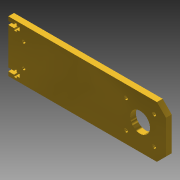
# Autodesk Inventor part: tiltColumnStepperSide02_RB01
Saved by Autodesk Inventor 2013 (Build 170138000, 138)
## iProperties
Created: 2014-06-14
Part Number: tiltColumnStepperSide02_RB01
Material: Gold
Document SubType Name: Modeling
Designer: Byron
Density: 19.3 g/cm^3
Mass: 1131.92 g
Surface Area: 227.905 cm^2
Volume: 58.6488 cm^3
Author: Byron
Autodesk Inventor part; units mm, degrees
ref_plane "YZ Plane" through (0, 0, 0) normal (1, 0, 0) x (0, 1, 0)
ref_plane "XZ Plane" through (0, 0, 0) normal (0, 1, 0) x (-1, 0, 0)
ref_plane "XY Plane" through (0, 0, 0) normal (0, 0, 1) x (1, 0, 0)
sketch "Sketch1" plane through (0, 0, 0) normal (0, 0, 1) x (1, 0, 0)
  circle A0 centre (15.5, -15.5) radius 2
  circle A1 centre (-15.5, -15.5) radius 2
  circle A2 centre (15.5, 15.5) radius 2
  circle A3 centre (-15.5, 15.5) radius 2
  line L0 (-21.15, 15.4985) -> (-15.4985, 21.15)
  line L1 (-15.4985, 21.15) -> (15.4985, 21.15)
  line L2 (15.4985, 21.15) -> (21.15, 15.4985)
  line L3 (21.15, 15.4985) -> (21.15, -15.4985)
  line L4 (21.15, -15.4985) -> (15.4985, -21.15)
  line L5 (15.4985, -21.15) -> (-15.4985, -21.15)
  line L6 (-15.4985, -21.15) -> (-21.15, -15.4985)
  line L7 (-21.15, -15.4985) -> (-21.15, 15.4985)
  line L8 (28.575, -18.574) -> (28.575, 18.574)
  line L9 (28.575, 18.574) -> (18.574, 28.575)
  line L10 (18.574, 28.575) -> (-18.574, 28.575)
  line L11 (-18.574, 28.575) -> (-28.575, 18.574)
  line L12 (-28.575, 18.574) -> (-28.575, -18.574)
  line L13 (-28.575, -18.574) -> (-18.574, -28.575)
  line L14 (-18.574, -28.575) -> (18.574, -28.575)
  line L15 (18.574, -28.575) -> (28.575, -18.574)
  line L16 (-18.574, -28.575) -> (-145.574, -28.575)
  line L17 (-145.574, -28.575) -> (-145.574, 28.575)
  line L18 (-145.574, 28.575) -> (-18.574, 28.575)
  line L19 (-18.574, 28.575) -> (-18.574, -28.575)
  circle A4 centre (0, 0) radius 11
  point P0 (0, 0)
  dimension "d0" = 127
  dimension "d1" = 57.15
  dimension "d2" = 57.15
  constraints: 40 end point, 5 centre point, 2 parallel, 1 horizontal, 1 perpendicular, 7 other
  measures "d0" distance of L17.end L18.end
  measures "d1" distance between parallel lines of L10 L14
  measures "d2" distance of L16.end L17.end
extrude "Extrusion1" add sketch "Sketch1" along normal blind 48.0547 contours L7 L6 L19 L13 L12 L11 L0 | L0 L19 L6 L7 | L19 L10 L9 L8 L15 L14 L6 L5 L4 L3 L2 L1 L0 | L0 L1 L2 L3 L4 L5 L6 L19 | L11 L12 L13 L16 L17 L18 | A4
sketch "Sketch2" plane through (0, 0, 0) normal (0, 0, -1) x (-1, 0, 0)
  line L0 (130.4486, -16.3493) -> (130.4486, -9.9993) projected
  line L1 (126.7402, -9.9993) -> (126.7402, -16.3493) projected
  line L2 (130.4486, 9.0507) -> (130.4486, 15.4007) projected
  line L3 (126.7402, 15.4007) -> (126.7402, 9.0507) projected
  line L4 (126.7402, -12.7) -> (130.4486, -12.7) construction
  line L5 (126.7402, 12.7) -> (130.4486, 12.7) construction
  circle A0 centre (128.5944, -12.7) radius 1.8542
  circle A1 centre (128.5944, 12.7) radius 1.8542
  dimension "d5" = 3.7084
  dimension "d6" = 3.7084
  constraints: 4 end point, 2 centre point
  measures "d5" diameter of A0
  measures "d6" diameter of A1
extrude "Extrusion2" cut sketch "Sketch2" against normal through all
sketch "Sketch3" plane through (0, 0, 0) normal (0, 0, -1) x (-1, 0, 0)
  line L0 (145.574, 28.575) -> (145.574, -28.575) projected
  line L1 (139.224, -24.0792) -> (145.574, -24.0792) projected
  line L2 (145.574, -28.575) -> (145.574, -24.0792) projected
  line L3 (-18.574, -28.575) -> (145.574, -28.575) projected
  line L4 (-28.575, -18.574) -> (-18.574, -28.575) projected
  line L5 (-28.575, 18.574) -> (-28.575, -18.574) projected
  line L6 (-18.574, 28.575) -> (-28.575, 18.574) projected
  line L7 (145.574, 28.575) -> (-18.574, 28.575) projected
  line L8 (145.574, 24.0792) -> (145.574, 28.575) projected
  line L9 (145.574, 24.0792) -> (139.224, 24.0792) projected
  line L10 (139.224, 24.0792) -> (139.224, 26.162) projected
  line L11 (139.224, 26.162) -> (136.43, 26.162) projected
  line L12 (136.43, 26.162) -> (136.43, 24.0792) projected
  line L13 (136.43, 24.0792) -> (132.874, 24.0792) projected
  line L14 (132.874, 24.0792) -> (132.874, 20.3708) projected
  line L15 (132.874, 20.3708) -> (136.43, 20.3708) projected
  line L16 (136.43, 20.3708) -> (136.43, 18.288) projected
  line L17 (136.43, 18.288) -> (139.224, 18.288) projected
  line L18 (139.224, 18.288) -> (139.224, 20.3708) projected
  line L19 (139.224, 20.3708) -> (145.574, 20.3708) projected
  line L20 (145.574, -20.3708) -> (145.574, 20.3708) projected
  line L21 (145.574, -20.3708) -> (139.224, -20.3708) projected
  line L22 (139.224, -20.3708) -> (139.224, -18.288) projected
  line L23 (139.224, -18.288) -> (136.43, -18.288) projected
  line L24 (136.43, -18.288) -> (136.43, -20.3708) projected
  line L25 (136.43, -20.3708) -> (132.874, -20.3708) projected
  line L26 (132.874, -20.3708) -> (132.874, -24.0792) projected
  line L27 (132.874, -24.0792) -> (136.43, -24.0792) projected
  line L28 (136.43, -24.0792) -> (136.43, -26.162) projected
  line L29 (136.43, -26.162) -> (139.224, -26.162) projected
  line L30 (139.224, -26.162) -> (139.224, -24.0792) projected
  circle A0 centre (128.5944, 12.7) radius 1.8542 projected
  circle A1 centre (128.5944, -12.7) radius 1.8542 projected
  circle A2 centre (-15.5, -15.5) radius 2 projected
  circle A3 centre (15.5, -15.5) radius 2 projected
  circle A4 centre (-15.5, 15.5) radius 2 projected
  circle A5 centre (15.5, 15.5) radius 2 projected
  circle A6 centre (0, 0) radius 11 projected
extrude "Extrusion3" cut sketch "Sketch3" against normal through all contours L0 L19 L18 L17 L16 L15 L14 L13 L12 L11 L10 L9 | L0 L1 L30 L29 L28 L27 L26 L25 L24 L23 L22 L21
sketch "Sketch4" plane through (0, 0, 0) normal (0, 0, -1) x (-1, 0, 0)
  circle A0 centre (0, 0) radius 11 projected
  point P0 (0, 0)
extrude "Extrusion4" cut sketch "Sketch4" against normal through all
equation "\"d2\" = d1"
body "Solid1"
